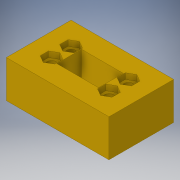
# Autodesk Inventor part: CapForCanBusConnector
Saved by Autodesk Inventor 2018.1 (Build 221171000, 171)
## iProperties
Created: 2017-10-25
Part Number: CapForCanBusConnector
Material: Generic
Document SubType Name: Modeling
Designer: steele
Density: 1 g/cm^3
Appearance: Gold
Author: steele
Autodesk Inventor part; units mm, degrees
ref_plane "YZ Plane" through (0, 0, 0) normal (1, 0, 0) x (0, 1, 0)
ref_plane "XZ Plane" through (0, 0, 0) normal (0, 1, 0) x (-1, 0, 0)
ref_plane "XY Plane" through (0, 0, 0) normal (0, 0, 1) x (1, 0, 0)
sketch "Sketch1" plane through (0, 0, 0) normal (0, 1, 0) x (-1, 0, 0)
  line L0 (18.6817, 11.7856) -> (-18.6817, 11.7856)
  line L1 (-18.6817, 11.7856) -> (-18.6817, -11.7856)
  line L2 (-18.6817, -11.7856) -> (18.6817, -11.7856)
  line L3 (18.6817, -11.7856) -> (18.6817, 11.7856)
  line L4 (18.6817, 11.7856) -> (-18.6817, -11.7856) construction
  line L5 (-18.6817, 11.7856) -> (18.6817, -11.7856) construction
  point P0 (0, 0)
  dimension "d0" = 37.3634
  dimension "d1" = 23.5712
  constraints: 12 end point, 2 midpoint, 2 parallel, 1 horizontal, 1 perpendicular
  measures "d0" distance of L1.end L2.end
  measures "d1" distance of L2.end L0.start
extrude "Extrusion1" add sketch "Sketch1" along normal blind 13.589
sketch "Sketch5" plane through (0, 0, 0) normal (0, -1, 0) x (1, 0, 0)
  line L0 (7.6073, 4.5085) -> (-7.6073, 4.5085)
  line L1 (-7.6073, 4.5085) -> (-7.6073, -4.5085)
  line L2 (-7.6073, -4.5085) -> (7.6073, -4.5085)
  line L3 (7.6073, -4.5085) -> (7.6073, 4.5085)
  line L4 (7.6073, 4.5085) -> (-7.6073, -4.5085) construction
  line L5 (-7.6073, 4.5085) -> (7.6073, -4.5085) construction
  point P0 (0, 0)
  dimension "d25" = 15.2146
  dimension "d26" = 9.017
  constraints: 12 end point, 2 midpoint, 2 parallel, 1 horizontal, 1 perpendicular
  measures "d25" distance of L1.end L2.end
  measures "d26" distance of L2.end L0.start
extrude "Extrusion3" cut sketch "Sketch5" against normal through all
sketch "Sketch8" plane through (0, 13.589, 0) normal (0, 1, 0) x (1, 0, 0)
  circle A0 centre (-10.4521, 3.556) radius 1.632 projected
  line L0 (-7.8168, 5.0775) -> (-7.8168, 2.0345)
  line L1 (-7.8168, 2.0345) -> (-10.4521, 0.5131)
  line L2 (-10.4521, 0.5131) -> (-13.0873, 2.0345)
  line L3 (-13.0873, 2.0345) -> (-13.0873, 5.0775)
  line L4 (-13.0873, 5.0775) -> (-10.4521, 6.5989)
  line L5 (-10.4521, 6.5989) -> (-7.8168, 5.0775)
  circle A1 centre (-10.4521, -3.556) radius 1.632 projected
  line L6 (-7.8169, -2.0345) -> (-7.8169, -5.0775)
  line L7 (-7.8169, -5.0775) -> (-10.4521, -6.5989)
  line L8 (-10.4521, -6.5989) -> (-13.0874, -5.0775)
  line L9 (-13.0874, -5.0775) -> (-13.0874, -2.0345)
  line L10 (-13.0874, -2.0345) -> (-10.4521, -0.5131)
  line L11 (-10.4521, -0.5131) -> (-7.8169, -2.0345)
  circle A2 centre (10.4521, -3.556) radius 1.632 projected
  line L12 (10.4521, -0.5131) -> (13.0873, -2.0345)
  line L13 (13.0873, -2.0345) -> (13.0873, -5.0775)
  line L14 (13.0873, -5.0775) -> (10.4521, -6.5989)
  line L15 (10.4521, -6.5989) -> (7.8168, -5.0775)
  line L16 (7.8168, -5.0775) -> (7.8168, -2.0345)
  line L17 (7.8168, -2.0345) -> (10.4521, -0.5131)
  circle A3 centre (10.4521, 3.556) radius 1.632 projected
  line L18 (13.0874, 5.0775) -> (13.0874, 2.0345)
  line L19 (13.0874, 2.0345) -> (10.4521, 0.5131)
  line L20 (10.4521, 0.5131) -> (7.8169, 2.0345)
  line L21 (7.8169, 2.0345) -> (7.8169, 5.0775)
  line L22 (7.8169, 5.0775) -> (10.4521, 6.5989)
  line L23 (10.4521, 6.5989) -> (13.0874, 5.0775)
  line L24 (18.6817, 11.7856) -> (-18.6817, 11.7856) construction
  line L25 (0, 11.7856) -> (0, -11.7856) construction
  line L26 (-18.6817, -11.7856) -> (18.6817, -11.7856) construction
  point P0 (0, 0)
  dimension "d43" = 5.2705
  constraints: 50 end point, 4 coincident, 4 parallel, 3 equal length, 2 midpoint, 52 other
  measures "d43" distance between parallel lines of L1 L4
extrude "Extrusion5" cut sketch "Sketch8" against normal blind 2.0955 contours A0 | L0 L1 L2 L3 L4 L5 | A1 | L6 L7 L8 L9 L10 L11 | A2 | L12 L13 L14 L15 L16 L17 | A3 | L18 L19 L20 L21 L22 L23
sketch "Sketch13" plane through (0, 11.4935, 0) normal (0, 1, 0) x (1, 0, 0)
  line L0 (-10.4521, 6.5989) -> (-7.8168, 5.0775) construction
  line L1 (-7.8169, -5.0775) -> (-10.4521, -6.5989) construction
  line L2 (-10.4521, 6.5989) -> (-10.4521, -6.5989) construction
  line L3 (10.4521, 6.5989) -> (13.0874, 5.0775) construction
  line L4 (10.4521, -6.5989) -> (7.8168, -5.0775) construction
  line L5 (10.4521, 6.5989) -> (10.4521, -6.5989) construction
  line L6 (-13.0873, 2.0345) -> (-13.0873, 5.0775) construction
  line L7 (-13.0873, 3.556) -> (13.0874, 3.556) construction
  line L8 (13.0874, 5.0775) -> (13.0874, 2.0345) construction
  line L9 (-13.0874, -5.0775) -> (-13.0874, -2.0345) construction
  line L10 (-13.0874, -3.556) -> (13.0873, -3.556) construction
  line L11 (13.0873, -2.0345) -> (13.0873, -5.0775) construction
  point P0 (0, 0)
  point P1 (-10.4521, 3.556)
  point P2 (10.4521, 3.556)
  point P3 (10.4521, -3.556)
  point P4 (-10.4521, -3.556)
  constraints: 8 end point, 8 point on line, 4 midpoint, 2 vertical
hole "Hole9" at (-10.4521, 11.4935, -3.556) at (10.4521, 11.4935, -3.556) at (10.4521, 11.4935, 3.556) at (-10.4521, 11.4935, 3.556) direction (0, -1, 0) diameter 3.302 end through all
equation "\"d0\" = PartWidth"
equation "\"d1\" = PartLength"
equation "\"d2\" = capHeight"
equation "\"d25\" = canWireHolderWidth + boardGap"
equation "\"d26\" = canWireHolderLength + boardGap"
equation "\"d43\" = hexNutWidth"
equation "\"d46\" = hexNutHeight"
equation "\"d76\" = boltHoleDiam"
equation "\"HoleWidth\" = 20.9042"
equation "\"HoleLength\" = 7.112"
equation "\"BaseOffset\" = 5.08"
equation "\"PartWidth\" = CanBaseWidth + 2 * BaseOffset"
equation "\"PartLength\" = CanBaseLength + 2 * BaseOffset"
equation "\"boardGap\" = 0.508"
equation "\"boltHeadHeight\" = 3.175"
equation "\"boltHeadDiam\" = 5.08"
equation "\"capHeight\" = 13.589"
equation "\"canWireHolderWidth\" = 14.7066"
equation "\"canWireHolderLength\" = 8.509"
equation "\"hexNutWidth\" = 5.2705"
equation "\"hexNutHeight\" = 2.0955"
equation "\"boltHoleDiam\" = 3.302"
equation "\"CanBaseWidth\" = 27.2034"
equation "\"CanBaseLength\" = 13.4112"
body "Solid1"
